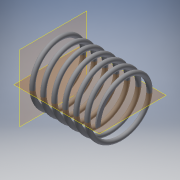
# Autodesk Inventor part: pruzina
Saved by Autodesk Inventor 2016 (Build 200138000, 138)
## iProperties
Created: 2016-11-29
Part Number: pruzina
Material: Generic
Document SubType Name: Modeling
Designer: Juraj
Density: 1 g/cm^3
Appearance: Default
Author: Juraj
Autodesk Inventor part; units mm, degrees
ref_plane "XZ Plane" through (0, 0, 0) normal (0, 1, 0) x (-1, 0, 0)
ref_plane "XY Plane" through (0, 0, 0) normal (0, 0, 1) x (1, 0, 0)
sketch "Sketch10" plane through (0, 0, 0) normal (1, 0, 0) x (0, 1, 0)
  circle A0 centre (0, 0) radius 8.3
  constraints: 1 centre point, 1 coincident
extrude "Extrusion6" add sketch "Sketch10" along normal blind 20
sketch "Sketch11" plane through (0, 0, 0) normal (0, 1, 0) x (-1, 0, 0)
  line L0 (-20, 8.3) -> (-20, -8.3) projected
  line L1 (-20, 0) -> (0, 0)
  circle A0 centre (-19.4, 7.7) radius 0.6
  dimension "d73" = 1.2
  constraints: 2 end point, 1 centre point, 1 horizontal, 1 midpoint, 1 tangent
  measures "d73" diameter of A0
coil "Coil5" sketch "Sketch11" operation intersect axis through (20, 0, 0) along (-1, 0, 0) pitch 4 turns 5 hand right
sketch "Sketch12" plane through (19.4, 0, 7.7) normal (0, -1, 0) x (1, 0, 0)
  circle A0 centre (0, 0) radius 0.6 projected
  circle A1 centre (0, 0) radius 0.6
  line L0 (0, -7.7) -> (8, -7.7)
  point P0 (-19.4, -7.7)
  point P1 (-0.6, 0)
  dimension "d74" = 8
  constraints: 2 end point, 1 centre point, 1 coincident, 1 horizontal, 1 horizontal alignment
  measures "d74" distance of L0.start L0.end
coil "Coil6" sketch "Sketch12" operation add axis through (19.4, 0, 0) along (1, 0, 0) pitch 1.5 turns 5.333333 hand right
ref_plane "Work Plane2" through (27.4, 0, 0) normal (1, 0, 0) x (0, 1, 0)
sketch "Sketch13" plane through (27.4, 0, 0) normal (1, 0, 0) x (0, 1, 0)
  line L0 (2.9838, 8.4803) -> (-8.742, 8.4803)
  line L1 (-8.742, 8.4803) -> (-8.742, -5.5139)
  line L2 (-8.742, -5.5139) -> (2.9838, -5.5139)
  line L3 (2.9838, -5.5139) -> (2.9838, 8.4803)
  point P0 (0, 0)
  constraints: 8 end point, 2 parallel, 1 horizontal, 1 perpendicular
extrude "Extrusion7" cut sketch "Sketch13" along normal blind 2
equation "\"d65\" = 0.2 * Vyska"
equation "\"d66\" = Vyska"
equation "\"d76\" = d74"
equation "\"Vyska\" = 20"
body "Solid3"
